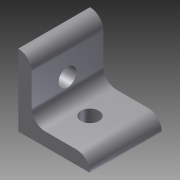
# Autodesk Inventor part: small L bracket
Saved by Autodesk Inventor 2012 (Build 160160000, 160)
## iProperties
Created: 2013-01-04
Part Number: small L bracket
Material: Default
Document SubType Name: Modeling
Designer: Bryce
Density: 1 g/cm^3
Author: Bryce
Autodesk Inventor part; units mm, degrees
ref_plane "YZ Plane" through (0, 0, 0) normal (1, 0, 0) x (0, 1, 0)
ref_plane "XZ Plane" through (0, 0, 0) normal (0, 1, 0) x (-1, 0, 0)
ref_plane "XY Plane" through (0, 0, 0) normal (0, 0, 1) x (1, 0, 0)
sketch "Sketch1" plane through (0, 0, 0) normal (0, 0, 1) x (1, 0, 0)
  line L0 (0, 0) -> (0, 25.4)
  line L1 (0, 0) -> (25.4, 0)
  line L2 (4.7625, 20.6375) -> (4.7625, 9.525)
  line L3 (9.525, 4.7625) -> (20.6375, 4.7625)
  arc A0 (4.7625, 20.6375) -> (0, 25.4) centre (0, 20.6375) ccw
  arc A1 (25.4, 0) -> (20.6375, 4.7625) centre (20.6375, 0) ccw
  arc A2 (4.7625, 9.525) -> (9.525, 4.7625) centre (9.525, 9.525) ccw
  dimension "d0" = 25.4
  dimension "d1" = 25.4
  dimension "d2" = 4.7625
  dimension "d3" = 4.7625
  constraints: 8 end point, 6 point on circle, 4 tangent, 3 centre point, 3 perpendicular, 2 point on line, 1 equal radius, 1 vertical
  measures "d0" distance of L0.start L0.end
  measures "d1" distance of L0.start L1.end
  measures "d2" distance between parallel lines of L0 L2
  measures "d3" distance between parallel lines of L1 L3
extrude "Extrusion1" add sketch "Sketch1" along normal blind 25.4
sketch "Sketch2" plane through (0, 0, 0) normal (0, -1, 0) x (1, 0, 0)
  line L0 (25.4, 25.4) -> (0, 25.4) projected
  line L1 (25.4, 0) -> (25.4, 25.4) projected
  circle A0 centre (12.7, 12.7) radius 3.175
  dimension "d6" = 6.35
  dimension "d7" = 12.7
  dimension "d8" = 12.7
  constraints: 1 centre point
  measures "d6" diameter of A0
  measures "d7" distance from line of L1 A0.centre
  measures "d8" distance from line of L0 A0.centre
extrude "Extrusion2" cut sketch "Sketch2" against normal blind 25.4
sketch "Sketch3" plane through (0, 0, 0) normal (-1, 0, 0) x (0, 0, 1)
  circle A0 centre (12.7, 12.7) radius 3.175
  dimension "d11" = 6.35
  constraints: 1 centre point
  measures "d11" diameter of A0
extrude "Extrusion3" cut sketch "Sketch3" against normal blind 25.4
equation "\"d3\" = d2"
body "Solid1"
